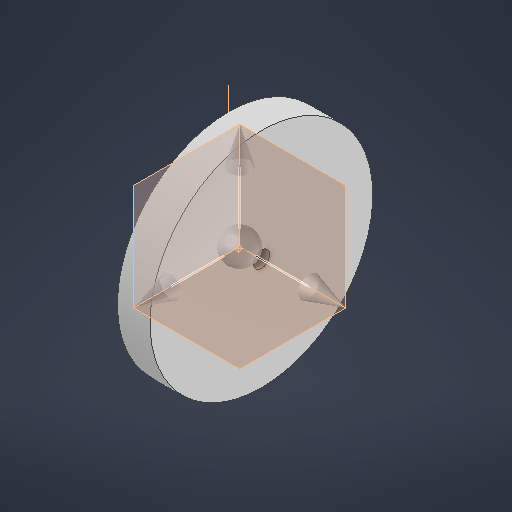
# Autodesk Inventor part: Vertical Spinner Weapon V3
Saved by Autodesk Inventor 2026.2 (Build 302298000, 298)
## iProperties
Created: 2023-08-18
Part Number: Vertical Spinner Weapon V3
Material: Generic
Document SubType Name: Modeling
Designer: vandj
Density: 1 g/cm^3
Appearance: Default
Mass: 70.3924 g
Surface Area: 175.698 cm^2
Volume: 70.3924 cm^3
Author: vandj
Autodesk Inventor part; units mm, degrees
ref_plane "YZ Plane" through (0, 0, 0) normal (1, 0, 0) x (0, 1, 0)
ref_plane "XZ Plane" through (0, 0, 0) normal (0, 1, 0) x (-1, 0, 0)
ref_plane "XY Plane" through (0, 0, 0) normal (0, 0, 1) x (1, 0, 0)
sketch "Sketch 1" plane through (0, 0, 0) normal (1, 0, 0) x (0, 1, 0)
  circle A0 centre (0, 0) radius 2.5
  circle A1 centre (0, 0) radius 25
  point P0 (1.2916, -31.2195)
  point P1 (0, 30.3272)
  point P2 (-0.1255, 30.3272)
  point P3 (0, -30.3272)
  point P4 (0.1231, -30.3272)
  point P5 (-1.2948, 31.2193)
  point P6 (0.0032, -40.9065)
  point P7 (0, -40.9065)
  point P8 (-1.4137, 30.3272)
  dimension "d22" = 5
  dimension "d51" = 50
  constraints: 2 centre point, 2 coincident
  measures "d22" diameter of A0
  measures "d51" diameter of A1
extrude "Interface" add sketch "Sketch 1" along normal blind 15
sketch "Sketch9" plane through (0, 0, 0) normal (-1, 0, 0) x (0, 0, 1)
  circle A0 centre (0, 0) radius 2.5 projected
  circle A1 centre (0, 0) radius 3.75
  dimension "d32" = 7.5
  constraints: 1 centre point, 1 coincident
  measures "d32" diameter of A1
extrude "Shaft Hole" cut sketch "Sketch9" against normal blind 28.1375
sketch "Sketch10" plane through (15, 0, 0) normal (1, 0, 0) x (0, 0, -1)
  circle A0 centre (0, 0) radius 3.75 projected
  circle A1 centre (0, 0) radius 7
  dimension "d35" = 14
  constraints: 1 centre point, 1 coincident
  measures "d35" diameter of A1
extrude "Bearing Hole" cut sketch "Sketch10" against normal blind 5
sketch "EDIT WEAPON SKETCH" plane through (0, 0, 0) normal (1, 0, 0) x (0, 1, 0)
  line L0 (80.6762, 135.1886) -> (80.6762, 42.6083) construction
  line L1 (80.6762, 42.6083) -> (64.461, 42.6083) construction
  line L2 (64.461, 42.6083) -> (64.461, 135.1886) construction
  line L3 (64.461, 135.1886) -> (80.6762, 135.1886) construction
  circle A0 centre (0, 0) radius 3.75 projected
  line L4 (0, 42.6083) -> (0, 40.7193)
  arc A1 (0.1376, 3.7475) -> (0, 0) centre (183.156, -4.8488) ccw
  arc A2 (0, 0) -> (0.1376, -3.7475) centre (183.156, 4.8488) ccw
  arc A3 (0, 0) -> (-0.1376, 3.7475) centre (-183.156, -4.8488) ccw
  circle A4 centre (0, 0) radius 51.2378
  point P0 (-10.4253, 109.8912)
  point P1 (22.8373, 112.0979)
  point P2 (30.5719, 96.5796)
  constraints: 9 point on circle, 4 centre point, 2 end point, 1 coincident, 1 point on line, 1 symmetric about line, 1 vertical, 2 other
extrude "EDIT WEAPON SHAPE" add sketch "EDIT WEAPON SKETCH" along normal up to surface (15 mm away)
sketch "Sketch12" plane through (0, 0, 0) normal (-1, 0, 0) x (0, 0, 1)
  point P0 (0, 0)
body "Solid1"
